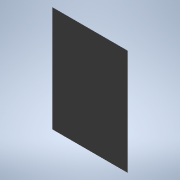
# Autodesk Inventor part: CONTROL_OPZETSTUK
Saved by Autodesk Inventor 2020 (Build 240168000, 168)
## iProperties
Created: 2020-06-03
Part Number: CONTROL_OPZETSTUK
Material: Generic
Document SubType Name: Sheet Metal
Designer: Gebruiker
Density: 1 g/cm^3
Sheet Metal Rule: Default_mm
Appearance: Default
Author: Gebruiker
Autodesk Inventor part; units mm, degrees
ref_plane "YZ Plane" through (0, 0, 0) normal (1, 0, 0) x (0, 1, 0)
ref_plane "XZ Plane" through (0, 0, 0) normal (0, 1, 0) x (-1, 0, 0)
ref_plane "XY Plane" through (0, 0, 0) normal (0, 0, 1) x (1, 0, 0)
sketch "Sketch1" plane through (0, 0, 0) normal (0, 0, 1) x (1, 0, 0)
  line L0 (-123.5, -173.5) -> (123.5, -173.5)
  line L1 (123.5, -173.5) -> (123.5, 173.5)
  line L2 (123.5, 173.5) -> (-123.5, 173.5)
  line L3 (-123.5, 173.5) -> (-123.5, -173.5)
  line L4 (-123.5, -173.5) -> (123.5, 173.5) construction
  line L5 (123.5, -173.5) -> (-123.5, 173.5) construction
  point P0 (0, 0)
  dimension "d0" = 247
  dimension "d1" = 347
  measures "d0" distance of L2.end L1.end
  measures "d1" distance of L1.end L0.end
extrude "Plate1" add sketch "Sketch1" along normal blind 0.5
equation "\"d2\" = Thickness"
equation "\"BendRadius\" = Thickness"
equation "\"BendReliefWidth\" = Thickness"
equation "\"BendReliefDepth\" = 0.5 * Thickness"
equation "\"CornerReliefSize\" = 4 * Thickness"
equation "\"MinimumRemnant\" = 2 * Thickness"
equation "\"TransitionRadius\" = BendRadius"
equation "\"JacobiRadiusSize\" = BendRadius"
equation "\"GapSize\" = Thickness"
equation "\"Thickness\" = 0.5"
body "Solid1"
